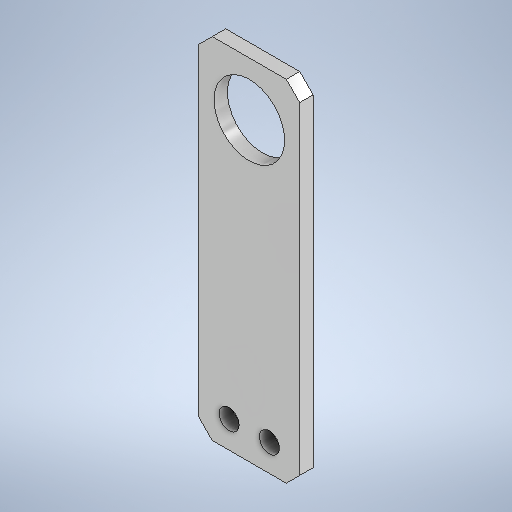
# Autodesk Inventor part: Loadcell_lever
Saved by Autodesk Inventor 2025.2 (Build 292293000, 293)
## iProperties
Created: 2026-07-22
Part Number: Loadcell_lever
Material: Generic
Document SubType Name: Modeling
Designer: Simon
Density: 1 g/cm^3
Appearance: Aluminum - Polished
Author: Simon
Autodesk Inventor part; units mm, degrees
ref_plane "YZ Plane" through (0, 0, 0) normal (1, 0, 0) x (0, 1, 0)
ref_plane "XZ Plane" through (0, 0, 0) normal (0, 1, 0) x (-1, 0, 0)
ref_plane "XY Plane" through (0, 0, 0) normal (0, 0, 1) x (1, 0, 0)
sketch "Sketch1" plane through (0, 0, 0) normal (0, 0, 1) x (1, 0, 0)
  line L0 (-7.5, -26) -> (7.5, -26)
  line L1 (7.5, -26) -> (7.5, 26)
  line L2 (7.5, 26) -> (-7.5, 26)
  line L3 (-7.5, 26) -> (-7.5, -26)
  line L4 (-7.5, -26) -> (7.5, 26) construction
  line L5 (7.5, -26) -> (-7.5, 26) construction
  line L6 (0, 26) -> (0, 18)
  circle A0 centre (0, 18) radius 5.25
  line L7 (0, -26) -> (0, -22)
  line L8 (-3, -22) -> (3, -22)
  circle A1 centre (-3, -22) radius 1.5
  circle A2 centre (3, -22) radius 1.5
  point P0 (0, 0)
  dimension "d0" = 15
  dimension "d1" = 52
  dimension "d2" = 8
  dimension "d3" = 10.5
  dimension "d6" = 4
  dimension "d7" = 6
  dimension "d8" = 3
  dimension "d9" = 3
  constraints: 18 end point, 5 midpoint, 3 centre point, 3 coincident, 3 parallel, 2 horizontal, 1 perpendicular, 1 vertical
  measures "d0" distance of L2.end L1.end
  measures "d1" distance of L1.end L0.end
  measures "d2" distance of L6.start L6.end
  measures "d3" diameter of A0
  measures "d6" distance of L7.start L7.end
  measures "d7" distance of L8.start L8.end
  measures "d8" diameter of A1
  measures "d9" diameter of A2
extrude "Extrusion1" add sketch "Sketch1" against normal blind 2
chamfer "Chamfer1" distance 2 angle 45 4 edges at (7.5, 26, -1) (-7.5, 26, -1) (7.5, -26, -1) (-7.5, -26, -1)
body "Solid1"
